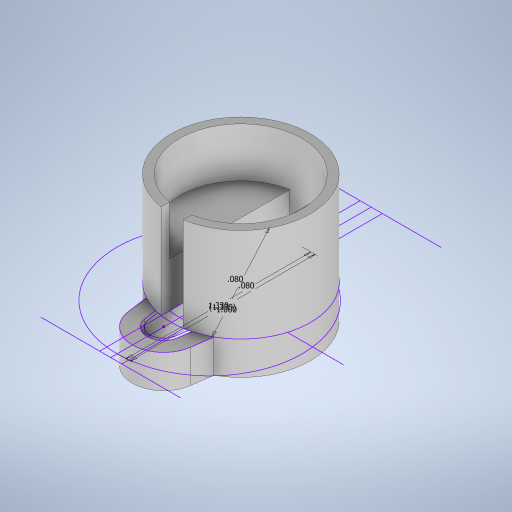
# Autodesk Inventor part: Servo Adapter 4
Saved by Autodesk Inventor 2024 (Build 280153000, 153)
## iProperties
Created: 2023-02-08
Part Number: Servo Adapter 4
Material: Generic
Document SubType Name: Modeling
Designer: tommy
Density: 1 g/cm^3
Appearance: Default
Author: tommy
Autodesk Inventor part; units mm, degrees
ref_plane "YZ Plane" through (0, 0, 0) normal (1, 0, 0) x (0, 1, 0)
ref_plane "XZ Plane" through (0, 0, 0) normal (0, 1, 0) x (-1, 0, 0)
ref_plane "XY Plane" through (0, 0, 0) normal (0, 0, 1) x (1, 0, 0)
sketch "Block1" plane through (0, 0, 0) normal (0, 0, 1) x (1, 0, 0)
  arc A0 (4.4042, -0.6007) -> (-4.4042, -0.6007) centre (0, 0) ccw
  arc A1 (-2.5167, -14.4402) -> (2.5167, -14.4402) centre (0, -14.097) ccw
  line L0 (-2.5167, -14.4402) -> (-4.4042, -0.6007)
  line L1 (4.4042, -0.6007) -> (2.5167, -14.4402)
  line L2 (-7.5501, -1.0297) -> (-5.6626, -14.8693)
  arc A2 (-5.6626, -14.8693) -> (5.6626, -14.8693) centre (0, -14.097) ccw
  line L3 (5.6626, -14.8693) -> (7.5501, -1.0297)
  arc A3 (7.5501, -1.0297) -> (-7.5501, -1.0297) centre (0, 0) ccw
  line L4 (-4.9018, -0.6685) -> (-3.0142, -14.5081)
  arc A4 (-3.0142, -14.5081) -> (3.0142, -14.5081) centre (0, -14.097) ccw
  line L5 (3.0142, -14.5081) -> (4.9018, -0.6685)
  arc A5 (4.9018, -0.6685) -> (-4.9018, -0.6685) centre (0, 0) ccw
  point P0 (0, -7.4025)
  dimension "d127" = 8.89
  dimension "d131" = 5.08
  dimension "d140" = 3.175
  measures "d127" diameter of A0
  measures "d131" diameter of A1
  measures "d140" distance between parallel lines of L0 L2
sketch "Sketch10" plane through (0, 0, 0) normal (0, 1, 0) x (-1, 0, 0)
  circle A0 centre (0, 0) radius 8.636
  line L0 (0, -14.097) -> (0, 0)
  arc A1 (-4.826, 10.0803) -> (-4.826, -10.0803) centre (0, 0) ccw
  circle A2 centre (0, 0) radius 11.176
  circle A3 centre (0, 0) radius 12.7
  line L1 (-12.7635, 23.7871) -> (12.7635, 23.7871)
  line L2 (0, 23.7871) -> (0, -23.7871)
  line L3 (-12.7635, -23.7871) -> (12.7635, -23.7871)
  line L4 (-2.032, 23.7871) -> (-2.032, -23.7871)
  line L5 (2.032, 23.7871) -> (2.032, -23.7871)
  line L6 (0, 11.176) -> (0, -22.606)
  line L7 (0, 11.176) -> (0, -22.606)
  circle A4 centre (0, -5.715) radius 16.891
  line L8 (0, -3.683) -> (-22.4394, -3.683)
  arc A5 (4.4042, -0.6007) -> (-4.4042, -0.6007) centre (0, 0) ccw
  arc A6 (-2.5167, -14.4402) -> (2.5167, -14.4402) centre (0, -14.097) ccw
  line L9 (-2.5167, -14.4402) -> (-4.4042, -0.6007)
  line L10 (4.4042, -0.6007) -> (2.5167, -14.4402)
  line L11 (-7.5501, -1.0297) -> (-5.6626, -14.8693)
  arc A7 (-5.6626, -14.8693) -> (5.6626, -14.8693) centre (0, -14.097) ccw
  line L12 (5.6626, -14.8693) -> (7.5501, -1.0297)
  arc A8 (7.5501, -1.0297) -> (-7.5501, -1.0297) centre (0, 0) ccw
  line L13 (-4.9018, -0.6685) -> (-3.0142, -14.5081)
  arc A9 (-3.0142, -14.5081) -> (3.0142, -14.5081) centre (0, -14.097) ccw
  line L14 (3.0142, -14.5081) -> (4.9018, -0.6685)
  arc A10 (4.9018, -0.6685) -> (-4.9018, -0.6685) centre (0, 0) ccw
  point P0 (2.032, -10.9897)
  point P1 (2.032, -12.5364)
  point P2 (-2.032, -12.5364)
  point P3 (-2.032, -10.9897)
  point P4 (-2.032, 10.9897)
  point P5 (2.032, 10.9897)
  point P6 (-6.1771, -11.0965)
  point P7 (6.1771, -11.0965)
  point P8 (6.4453, -9.1302)
  point P9 (7.0009, -5.0565)
  point P10 (2.032, 8.3935)
  point P11 (-2.032, 8.3935)
  point P12 (-7.0009, -5.0565)
  point P13 (-6.4453, -9.1302)
  point P14 (6.1771, -11.0965)
  point P15 (-6.1771, -11.0965)
  point P16 (2.032, 7.3441)
  point P17 (-7.0009, -5.0565)
  point P18 (7.0009, -5.0565)
  point P19 (6.4453, -9.1302)
  point P20 (2.032, -19.4386)
  point P21 (-6.4453, -9.1302)
  point P22 (2.032, -8.3935)
  point P23 (-2.032, 7.3441)
  point P24 (-2.032, -19.4386)
  point P25 (-2.032, -8.3935)
  point P26 (6.1771, -11.0965)
  point P27 (-6.1771, -11.0965)
  point P28 (2.032, 7.3441)
  point P29 (-7.0009, -5.0565)
  point P30 (7.0009, -5.0565)
  point P31 (6.4453, -9.1302)
  point P32 (2.032, -19.4386)
  point P33 (-6.4453, -9.1302)
  point P34 (-2.032, 7.3441)
  point P35 (-2.032, -19.4386)
  point P36 (-6.4453, -9.1302)
  dimension "d149" = 25.4
  dimension "d148" = 2.032
  dimension "d147" = 2.032
  dimension "d146" = 33.782
  dimension "d159" = 33.782
  constraints: 18 end point, 4 centre point, 4 point on circle, 3 coincident, 3 equal length, 3 midpoint, 2 point on line, 1 vertical, 1 vertical alignment, 4 other
  measures "d149" diameter of A3
  measures "d148" distance between parallel lines of L2 L4
  measures "d147" distance between parallel lines of L2 L5
  measures "d146" distance of L6.start L6.end
  measures "d159" distance of L6.start L6.end
extrude "Extrusion21" add sketch "Sketch10" against normal blind 17.145 contours L5 A4 A3 L12 A2 | A2 A4 L5 | L12 A3 L14 A2 | A4 L4 A3 L2 | L2 A3 L5 A4 | A2 L4 A4 | L5 A3 A4 | L14 A3 L10 A2 | A2 A1 L8 A3 A4 L4 | A4 A3 L4 | L10 A3 L5 A2 | A1 L11 A3 L8 | A1 A2 L13 A3 L11 | A2 L9 A3 L13 | L4 A3 L9 A2
extrude "Extrusion22" add sketch "Sketch10" against normal blind 8.128 contours A0 L12 A8 L5 | A0 L5 A2 L12 | L12 A2 L14 A0 | A0 L14 A10 L5 A8 L12 | L14 A2 L10 A0 | A0 L10 A5 L5 A10 L14 | L4 A8 L11 L8 A0 | A0 L8 A1 A2 L4 | L10 A2 L5 A0 | A0 L5 A5 L10 | L8 L11 A0 | A0 L11 A1 L8 | L4 A10 L13 L8 L11 A8 | L11 L8 L13 A0 | A0 L13 A2 A1 L11 | L4 A5 L9 L8 L13 A10 | L13 L8 L9 A0 | A0 L9 A2 L13 | L4 L8 L9 A5 | L4 A2 L9 A0 | A0 L9 L8 L4
extrude "Extrusion23" add sketch "Sketch10" along normal blind 6.096 contours A0 L12 A8 L5 | L5 A8 L2 A0 | A0 L2 A2 L5 | L12 A2 L14 A0 | A0 L14 A10 L5 A8 L12 | L2 A8 L4 A0 | A0 L4 A2 L2 | L5 A4 A3 L12 A2 | A2 A4 L5 | L5 A10 L2 A8 | L14 A2 L10 A0 | A0 L10 A5 L5 A10 L14 | L12 A3 L14 A2 | L4 A8 L11 L8 A0 | A4 L4 A3 L2 | L2 A3 L5 A4 | A2 L4 A4 | L2 A10 L4 A8 | L5 A3 A4 | L5 A5 L2 A10 | L14 A3 L10 A2 | L12 A7 L5 A9 L14 A3 | L8 L11 A0 | A2 A1 L8 A3 A4 L4 | L4 A10 L13 L8 L11 A8 | A4 A3 L4 | L2 A5 L4 A10 | L14 A9 L5 A6 L10 A3 | L11 L8 L13 A0 | A0 L13 A2 A1 L11 | A1 L11 A3 L8 | L4 A5 L9 L8 L13 A10 | A7 L2 A9 L5 | L13 L8 L9 A0 | A0 L9 A2 L13 | A1 A2 L13 A3 L11 | A9 L2 A6 L5 | A7 L4 A9 L2 | A2 L9 A3 L13 | A3 L13 A9 L4 A7 L11 | A9 L4 A6 L2 | A3 L9 A6 L4 A9 L13
extrude "Extrusion24" cut sketch "Sketch10" along normal blind 6.096 contours L14 A2 L10 A0 | A0 L10 A5 L5 A10 L14 | L5 A5 L2 A10 | L10 A2 L5 A0 | A0 L5 A5 L10 | L14 A3 L10 A2 | L2 A5 L4 A10 | L5 A0 L0 L2 A5 | L5 A2 L0 A0 | L10 A3 L5 A2 | L14 A9 L5 A6 L10 A3 | L4 A5 L9 L8 L13 A10 | L2 L0 L8 L4 A5 | L0 A2 L4 A0 | A0 L4 L8 L0 | L5 A3 L0 A2 | L10 A6 L5 A3 | L13 L8 L9 A0 | A0 L9 A2 L13 | L4 L8 L9 A5 | L4 A2 L9 A0 | A0 L9 L8 L4 | L0 A3 L4 A2 | L5 A6 L2 L0 A3 | A9 L2 A6 L5 | A2 L9 A3 L13 | L4 A3 L9 A2 | L0 L2 A6 L4 A3 | A9 L4 A6 L2 | A3 L9 A6 L4 A9 L13 | L4 A6 L9 A3
body "Solid1"
